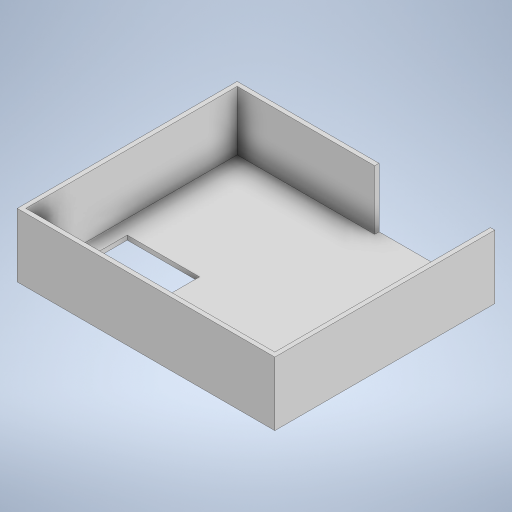
# Autodesk Inventor part: back side
Saved by Autodesk Inventor 2023 (Build 270158030, 158C)
## iProperties
Created: 2023-03-06
Part Number: back side
Material: Generic
Document SubType Name: Modeling
Designer: fatih
Density: 1 g/cm^3
Appearance: Default
Author: fatih
Autodesk Inventor part; units mm, degrees
ref_plane "YZ Plane" through (0, 0, 0) normal (1, 0, 0) x (0, 1, 0)
ref_plane "XZ Plane" through (0, 0, 0) normal (0, 1, 0) x (-1, 0, 0)
ref_plane "XY Plane" through (0, 0, 0) normal (0, 0, 1) x (1, 0, 0)
sketch "Sketch1" plane through (0, 0, 0) normal (0, 1, 0) x (-1, 0, 0)
  line L0 (0, 0) -> (178, 0)
  line L1 (178, 0) -> (178, -152)
  line L2 (178, -152) -> (0, -152)
  line L3 (0, -152) -> (0, 0)
  dimension "d1" = 152
  dimension "d2" = 178
  constraints: 8 end point, 2 parallel, 1 horizontal, 1 perpendicular
  measures "d1" distance of L0.end L1.end
  measures "d2" distance of L0.start L0.end
extrude "Extrusion1" add sketch "Sketch1" along normal blind 44
shell "Shell1" thickness 3 removed faces 1 at (-118.6667, 44, -101.3333)
sketch "Sketch3" plane through (0, 0, -152) normal (0, 0, -1) x (-1, 0, 0)
  line L0 (3, 3) -> (3, 44) projected
  line L1 (0, 44) -> (178, 44) projected
  line L2 (3, 3) -> (80, 3)
  line L3 (80, 3) -> (80, 44)
  line L4 (80, 44) -> (3, 44)
  line L5 (3, 44) -> (3, 3)
  point P0 (0, 0)
  dimension "d9" = 77
  constraints: 8 end point, 2 parallel, 1 horizontal, 1 perpendicular, 1 point on line
  measures "d9" distance of L4.end L3.end
extrude "Extrusion3" cut sketch "Sketch3" against normal blind 4
sketch "Sketch4" plane through (0, 0, 0) normal (0, -1, 0) x (1, 0, 0)
  line L0 (-175, -3) -> (-175, -149) projected
  line L1 (-175, -3) -> (-165, -3)
  line L2 (-165, -3) -> (-165, -13)
  line L3 (-165, -13) -> (-175, -13)
  line L4 (-175, -13) -> (-175, -3)
  line L5 (-165, -13) -> (-115, -13)
  line L6 (-115, -13) -> (-115, -63)
  line L7 (-115, -63) -> (-165, -63)
  line L8 (-165, -63) -> (-165, -13)
  point P0 (0, 0)
  dimension "d12" = 10
  dimension "d13" = 10
  dimension "d14" = 50
  dimension "d15" = 50
  constraints: 16 end point, 4 parallel, 2 horizontal, 2 perpendicular
  measures "d12" distance of L2.end L3.end
  measures "d13" distance of L1.end L2.end
  measures "d14" distance of L6.end L7.end
  measures "d15" distance of L5.end L6.end
extrude "Extrusion4" cut sketch "Sketch4" against normal blind 4 contours L5 L6 L7 L8
body "Solid1"
